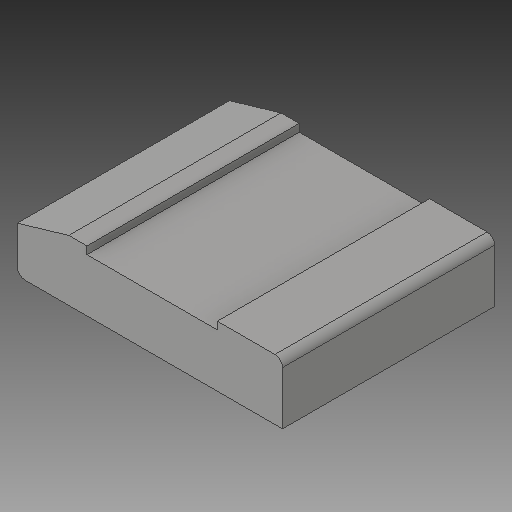
# Autodesk Inventor part: lift holder
Saved by Autodesk Inventor 2019 (Build 230136000, 136)
## iProperties
Created: 2018-10-20
Part Number: lift holder
Material: PC/ABS Plastic
Document SubType Name: Modeling
Designer: User
Density: 0.357273 g/cm^3
Appearance: Orange
Author: User
Autodesk Inventor part; units mm, degrees
ref_plane "YZ Plane" through (0, 0, 0) normal (1, 0, 0) x (0, 1, 0)
ref_plane "XZ Plane" through (0, 0, 0) normal (0, 1, 0) x (-1, 0, 0)
ref_plane "XY Plane" through (0, 0, 0) normal (0, 0, 1) x (1, 0, 0)
sketch "Sketch1" plane through (0, 0, 0) normal (0, 1, 0) x (-1, 0, 0)
  line L0 (0, 0) -> (111.125, 0)
  line L1 (111.125, 0) -> (111.125, -88.9)
  line L2 (111.125, -88.9) -> (0, -88.9)
  line L3 (0, -88.9) -> (0, 0)
  dimension "d0" = 111.125
  dimension "d1" = 88.9
  constraints: 8 end point, 2 parallel, 1 horizontal, 1 perpendicular
  measures "d0" distance of L1.end L2.end
  measures "d1" distance of L0.end L1.end
extrude "Extrusion1" add sketch "Sketch1" along normal blind 25.4
sketch "Sketch2" plane through (0, 25.4, 0) normal (0, 1, 0) x (1, 0, 0)
  line L0 (0, 88.9) -> (-111.125, 88.9) projected
  line L1 (-111.125, 0) -> (0, 0) projected
  line L2 (-27.305, 88.9) -> (-81.915, 88.9)
  line L3 (-81.915, 88.9) -> (-81.915, 0)
  line L4 (-81.915, 0) -> (-27.305, 0)
  line L5 (-27.305, 0) -> (-27.305, 88.9)
  line L6 (0, 0) -> (0, 88.9) projected
  dimension "d4" = 111.125
  dimension "d5" = 54.61
  dimension "d6" = 27.305
  constraints: 8 end point, 2 parallel, 2 point on line, 1 horizontal, 1 perpendicular
  measures "d4" distance of L1.start L1.end
  measures "d5" distance between parallel lines of L5 L3
  measures "d6" distance between parallel lines of L6 L5
extrude "Extrusion2" cut sketch "Sketch2" against normal blind 3.175 contours L5 L1 L3 L0
sketch "Sketch4" plane through (-111.125, 0, 0) normal (0, 0, 1) x (1, 0, 0)
  line L0 (0, 0) -> (0, 25.4) projected
  line L1 (0, 19.05) -> (21.59, 25.4)
  line L2 (0, 25.4) -> (29.21, 25.4) projected
  point P0 (111.125, 0)
  dimension "d17" = 6.35
  dimension "d18" = 7.62
  constraints: 2 end point, 2 point on line
  measures "d17" distance from line of L1.start L2
  measures "d18" distance of L2.end L1.end
extrude "Extrusion4" cut sketch "Sketch4" against normal through all
fillet "Fillet2" radius 3.175 2 edges at (-111.125, 0, -44.45) (0, 25.4, -44.45)
body "Solid1"
